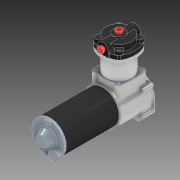
# Autodesk Inventor part: 215 Thomas Compressor
Saved by Autodesk Inventor 2022 (Build 260153000, 153)
## iProperties
Created: 2021-07-29
Part Number: 215 Thomas Compressor
Material: Generic
Document SubType Name: Modeling
Designer: kevin
Density: 1 g/cm^3
Appearance: Default
Author: kevin
Autodesk Inventor part; units mm, degrees
ref_plane "YZ Plane" through (0, 0, 0) normal (1, 0, 0) x (0, 1, 0)
sketch "Sketch37" plane through (0, 0, 0) normal (1, 0, 0) x (0, 1, 0)
  line L0 (0, 0) -> (27.7812, 0)
  line L1 (27.7812, 0) -> (27.7812, 50.8)
  line L2 (27.7812, 50.8) -> (25.4, 50.8)
  line L3 (25.4, 50.8) -> (25.4, 136.271)
  line L4 (25.4, 136.271) -> (15.5575, 136.271)
  line L5 (15.5575, 136.271) -> (15.5575, 138.811)
  line L6 (15.5575, 138.811) -> (12.7, 138.811)
  line L7 (12.7, 138.811) -> (8.2867, 146.431)
  line L8 (8.2867, 146.431) -> (0, 146.431)
  line L9 (0, 146.431) -> (0, 0)
  line L10 (0, 133.096) -> (25.4, 133.096)
  line L11 (25.4, 50.8) -> (0, 50.8)
  dimension "d151" = 27.7812
  dimension "d152" = 25.4
  dimension "d153" = 15.5575
  dimension "d154" = 12.7
  dimension "d156" = 8.2867
  dimension "d157" = 85.471
  dimension "d158" = 50.8
  dimension "d159" = 2.54
  dimension "d160" = 7.62
  dimension "d172" = 3.175
  constraints: 24 end point, 8 perpendicular, 3 point on line, 1 collinear, 1 horizontal, 1 parallel
  measures "d151" distance between parallel lines of L9 L1
  measures "d152" distance between parallel lines of L9 L3
  measures "d153" distance between parallel lines of L9 L5
  measures "d154" distance from line of L9 L6.end
  measures "d156" distance of L7.end L8.end
  measures "d157" distance of L2.end L3.end
  measures "d158" distance of L0.end L1.end
  measures "d159" distance of L4.end L5.end
  measures "d160" distance between parallel lines of L6 L8
  measures "d172" distance between parallel lines of L10 L4
revolve "Revolution1" add sketch "Sketch37" angle 360 about axis through (0, 0, 146.431) along (0, 0, -1) contours L9 L11 L2 L1 L0
sketch "Sketch38" plane through (0, 0, 0) normal (0, 1, 0) x (-1, 0, 0)
  line L0 (-17.4625, 42.8625) -> (17.4625, 42.8625) construction
  line L1 (17.4625, 42.8625) -> (17.4625, 7.9375) construction
  line L2 (17.4625, 7.9375) -> (-17.4625, 7.9375)
  line L3 (-17.4625, 7.9375) -> (-17.4625, 42.8625) construction
  line L4 (-17.4625, 42.8625) -> (17.4625, 7.9375) construction
  line L5 (17.4625, 42.8625) -> (-17.4625, 7.9375) construction
  circle A0 centre (0, 25.4) radius 20.6375
  line L6 (17.4625, 42.8625) -> (17.4625, 7.9375) construction
  line L7 (12.3825, 42.8625) -> (12.3825, 7.9375) construction
  line L8 (22.5425, 7.9375) -> (22.5425, 42.8625)
  arc A1 (22.5425, 42.8625) -> (12.3825, 42.8625) centre (17.4625, 42.8625) ccw
  arc A2 (12.3825, 7.9375) -> (22.5425, 7.9375) centre (17.4625, 7.9375) ccw
  line L9 (-17.4625, 7.9375) -> (-17.4625, 42.8625) construction
  line L10 (-12.3825, 7.9375) -> (-12.3825, 42.8625) construction
  line L11 (-22.5425, 42.8625) -> (-22.5425, 7.9375)
  arc A3 (-22.5425, 7.9375) -> (-12.3825, 7.9375) centre (-17.4625, 7.9375) ccw
  arc A4 (-12.3825, 42.8625) -> (-22.5425, 42.8625) centre (-17.4625, 42.8625) ccw
  line L12 (-27.7813, 50.8) -> (27.7813, 50.8) construction
  line L13 (17.4625, 42.8625) -> (13.056, 45.3901) construction
  line L14 (-13.056, 45.3901) -> (13.056, 45.3901) construction
  line L15 (-17.4625, 42.8625) -> (-13.056, 45.3901) construction
  arc A5 (13.056, 45.3901) -> (-13.056, 45.3901) centre (0, 12.9973) ccw
  line L16 (27.7812, 50.8) -> (27.7812, 0) construction
  line L17 (27.7812, 25.4) -> (-27.7812, 25.4) construction
  line L18 (-27.7812, 50.8) -> (-27.7812, 0) construction
  circle A6 centre (-17.4625, 42.8625) radius 1.7272
  circle A7 centre (-17.4625, 7.9375) radius 1.7272
  circle A8 centre (17.4625, 7.9375) radius 1.7272
  circle A9 centre (17.4625, 42.8625) radius 1.7272
  arc A10 (-13.056, 5.4099) -> (13.056, 5.4099) centre (0, 37.8027) ccw
  point P0 (0, 0)
  point P1 (17.4625, 25.4)
  point P2 (-17.4625, 25.4)
  point P3 (0, 25.4)
  point P4 (12.3825, 7.9375)
  point P5 (13.056, 45.3901)
  point P6 (-13.056, 45.3901)
  point P7 (-12.3825, 7.9375)
  point P8 (-10.9985, 7.9375)
  point P9 (10.9985, 7.9375)
  point P10 (13.056, 5.4099)
  dimension "d162" = 34.925
  dimension "d163" = 41.275
  dimension "d164" = 10.16
  dimension "d165" = 25.4
  dimension "d166" = 5.08
  dimension "d167" = 34.925
  dimension "d168" = 23.876
  dimension "d169" = 3.4544
  constraints: 36 end point, 12 point on circle, 11 centre point, 8 equal length, 8 midpoint, 8 tangent, 5 coincident, 4 equal radius, 3 symmetric about line, 2 horizontal, 1 perpendicular, 1 other
  measures "d162" distance of L0.end L1.end
  measures "d163" diameter of A0
  measures "d164" distance between parallel lines of L11 L10
  measures "d165" distance from line of A0.centre L12
  measures "d166" distance of L0.end L13.end
  measures "d167" radius of A5
  measures "d168" distance of point (0, 25.4) L13.end
  measures "d169" diameter of A8
extrude "Extrusion4" add sketch "Sketch38" along normal blind 35.8775
revolve "Revolution2" add sketch "Sketch37" angle 360 about axis through (0, 0, 146.431) along (0, 0, -1) separate body contours L9 L8 L7 L6 L5 L4 L3 L10
revolve "Revolution3" add sketch "Sketch37" angle 360 about axis through (0, 0, 146.431) along (0, 0, -1) separate body contours L9 L10 L3 L11
sketch "Sketch39" plane through (0, 35.8775, 0) normal (0, 1, 0) x (1, 0, 0)
  circle A0 centre (17.4625, -7.9375) radius 1.7272 construction
  circle A1 centre (-17.4625, -42.8625) radius 1.7272 construction
  line L0 (17.4625, -7.9375) -> (-17.4625, -42.8625) construction
  circle A2 centre (0, -25.4) radius 20.6375
  point P0 (0, 0)
  dimension "d175" = 41.275
  constraints: 2 end point, 1 centre point, 1 midpoint
  measures "d175" diameter of A2
extrude "Extrusion5" add sketch "Sketch39" along normal blind 28.575 separate body
sketch "Sketch40" plane through (0, 64.4525, 25.4) normal (0, 1, 0) x (1, 0, 0)
  arc A0 (20.5522, -18.5984) -> (20.5522, 18.5984) centre (-12.7, 0) ccw
  arc A1 (20.5522, 18.5984) -> (18.5984, 20.5522) centre (16.1186, 16.1186) ccw
  arc A2 (18.5984, 20.5522) -> (-18.5984, 20.5522) centre (0, -12.7) ccw
  arc A3 (-18.5984, 20.5522) -> (-20.5522, 18.5984) centre (-16.1186, 16.1186) ccw
  arc A4 (-20.5522, 18.5984) -> (-20.5522, -18.5984) centre (12.7, 0) ccw
  arc A5 (-20.5522, -18.5984) -> (-18.5984, -20.5522) centre (-16.1186, -16.1186) ccw
  arc A6 (-18.5984, -20.5522) -> (18.5984, -20.5522) centre (0, 12.7) ccw
  arc A7 (18.5984, -20.5522) -> (20.5522, -18.5984) centre (16.1186, -16.1186) ccw
  circle A8 centre (0, 0) radius 20.6375
  circle A9 centre (17.4625, -17.4625) radius 1.7272 projected
  circle A10 centre (-17.4625, -17.4625) radius 1.7272 projected
  circle A11 centre (-17.4625, 17.4625) radius 1.7272 projected
  circle A12 centre (17.4625, 17.4625) radius 1.7272 projected
  line L0 (0, -12.7) -> (0, 0) construction
  line L1 (0, 0) -> (-12.7, 0) construction
  line L2 (0, 0) -> (12.7, 0) construction
  line L3 (0, 12.7) -> (0, 0) construction
  line L4 (-16.1186, -16.1186) -> (0, 0) construction
  line L5 (-16.1186, 16.1186) -> (0, 0) construction
  line L6 (16.1186, -16.1186) -> (0, 0) construction
  line L7 (0, 0) -> (16.1186, 16.1186) construction
  line L8 (-22.5425, 17.4625) -> (-22.5425, -17.4625) construction
  line L9 (-22.5425, 0) -> (22.5425, 0) construction
  line L10 (22.5425, 17.4625) -> (22.5425, -17.4625) construction
  line L11 (0, 25.4) -> (0, -25.4) construction
  line L12 (27.7813, -25.4) -> (-27.7812, -25.4) construction
  line L13 (27.7813, 25.4) -> (-27.7812, 25.4) construction
  dimension "d179" = 5.08
  dimension "d180" = 12.7
  dimension "d181" = 45
  dimension "d182" = 41.275
  dimension "d197" = 50.8
  constraints: 20 end point, 16 point on circle, 9 centre point, 6 equal radius, 5 tangent, 4 midpoint, 3 equal length, 3 perpendicular, 2 vertical, 1 collinear, 1 horizontal
  measures "d179" radius of A1
  measures "d180" distance of L0.end L1.end
  measures "d181" angle of L0 L4
  measures "d182" diameter of A8
  measures "d197" distance of L11.start L11.end
extrude "Extrusion6" add sketch "Sketch40" along normal blind 6.35 separate body contours A7 A6 A5 A4 A3 A2 A1 A0 | A8
sketch "Sketch41" plane through (0, 70.8025, 25.4) normal (0, 1, 0) x (1, 0, 0)
  circle A0 centre (0, 0) radius 20.6375 construction
  circle A1 centre (0, 0) radius 20.0025
  point P0 (0, 25.4)
  dimension "d185" = 40.005
  constraints: 1 centre point, 1 coincident
  measures "d185" diameter of A1
extrude "Extrusion7" add sketch "Sketch41" along normal blind 9.525 bodies 5
sketch "Sketch42" plane through (0, 80.3275, 25.4) normal (0, 1, 0) x (1, 0, 0)
  circle A0 centre (0, 0) radius 20.0025 projected
  circle A1 centre (0, 0) radius 9.144
  point P0 (0, 25.4)
  dimension "d188" = 18.288
  constraints: 1 centre point, 1 coincident
  measures "d188" diameter of A1
extrude "Extrusion8" add sketch "Sketch42" along normal blind 2.54 contours A1 bodies 5
sketch "Sketch43" plane through (0, 70.8025, 25.4) normal (0, 1, 0) x (1, 0, 0)
  line L0 (16.1186, -16.1186) -> (-16.1186, 16.1186) construction
  circle A0 centre (0, 0) radius 9.144 projected
  line L1 (19.7107, -12.5265) -> (-12.5265, 19.7107)
  line L2 (-19.7107, 12.5265) -> (12.5265, -19.7107)
  arc A1 (12.5265, -19.7107) -> (19.7107, -12.5265) centre (16.1186, -16.1186) ccw
  arc A2 (-12.5265, 19.7107) -> (-19.7107, 12.5265) centre (-16.1186, 16.1186) ccw
  line L3 (16.1186, 16.1186) -> (-16.1186, -16.1186) construction
  line L4 (19.7107, 12.5265) -> (-12.5265, -19.7107)
  line L5 (-19.7107, -12.5265) -> (12.5265, 19.7107)
  arc A3 (19.7107, 12.5265) -> (12.5265, 19.7107) centre (16.1186, 16.1186) ccw
  arc A4 (-19.7107, -12.5265) -> (-12.5265, -19.7107) centre (-16.1186, -16.1186) ccw
  arc A5 (-20.5522, -18.5984) -> (-18.5984, -20.5522) centre (-16.1186, -16.1186) ccw projected
  line L6 (-22.5425, 0) -> (22.5425, 0) construction
  circle A6 centre (-17.4625, -17.4625) radius 1.7272 projected
  circle A7 centre (-17.4625, 17.4625) radius 1.7272 projected
  circle A8 centre (17.4625, 17.4625) radius 1.7272 projected
  circle A9 centre (17.4625, -17.4625) radius 1.7272 projected
  circle A10 centre (0, 0) radius 9.144 projected
  circle A11 centre (0, 0) radius 20.0025 projected
  line L7 (22.5425, -17.4625) -> (22.5425, 17.4625) construction
  line L8 (-22.5425, 17.4625) -> (-22.5425, -17.4625) construction
  point P0 (0, 25.4)
  point P1 (-10.0881, -17.2723)
  point P2 (-17.2723, -10.0881)
  point P3 (-17.2723, 10.0881)
  point P4 (-10.0881, 17.2723)
  point P5 (10.0881, 17.2723)
  point P6 (17.2723, 10.0881)
  point P7 (17.2723, -10.0881)
  point P8 (10.0881, -17.2723)
  dimension "d191" = 10.16
  dimension "d192" = 45
  constraints: 18 end point, 9 tangent, 8 point on circle, 4 centre point, 4 midpoint, 2 parallel, 2 perpendicular, 1 equal radius
  measures "d191" distance between parallel lines of L4 L5
  measures "d192" angle of L6 L5
extrude "Extrusion9" add sketch "Sketch43" along normal blind 5.334 contours A11 L5 A3 L4 | L1 A1 L2 A11 | A11 L2 A2 L1 | L4 A4 L5 A11 bodies 5
ref_plane "Work Plane1" through (0, 64.4525, 0) normal (0, 0, -1) x (-1, 0, 0)
sketch "Sketch44" plane through (0, 64.4525, 0) normal (0, 0, -1) x (-1, 0, 0)
  line L0 (20.6375, 0) -> (-20.6375, 0) projected
  line L1 (0, 0) -> (0, 8.89) construction
  line L2 (8.89, 0) -> (8.89, 8.89)
  line L3 (-8.89, 8.89) -> (-8.89, 0)
  arc A0 (-8.89, 0) -> (8.89, 0) centre (0, 0) ccw
  arc A1 (8.89, 8.89) -> (-8.89, 8.89) centre (0, 8.89) ccw
  line L4 (9.144, 18.415) -> (-9.144, 18.415) projected
  point P0 (0, -64.4525)
  point P1 (0, 4.445)
  dimension "d195" = 17.78
  dimension "d196" = 9.525
  constraints: 8 end point, 4 point on circle, 4 tangent, 2 centre point, 2 midpoint, 1 parallel, 1 vertical
  measures "d195" distance between parallel lines of L2 L3
  measures "d196" distance from line of L4 L1.end
extrude "Extrusion10" add sketch "Sketch44" against normal blind 50.8 contours L0 L3 A1 L2 bodies 5
move or copy body "Move Body1" bodies to move or copy 5 copy no translate (0, 4.7625, 0)
sketch "Sketch45" plane through (12.7, 69.215, 25.4) normal (0, -1, 0) x (1, 0, 0)
  circle A0 centre (4.7625, 17.4625) radius 1.7272 projected
  circle A1 centre (4.7625, -17.4625) radius 1.7272 projected
  arc A2 (-21.59, 24.3483) -> (-31.2984, 20.5522) centre (-12.7, -12.7) ccw projected
  arc A3 (-31.2984, 20.5522) -> (-33.2522, 18.5984) centre (-28.8186, 16.1186) ccw projected
  arc A4 (-33.2522, 18.5984) -> (-33.2522, -18.5984) centre (0, 0) ccw projected
  arc A5 (-33.2522, -18.5984) -> (-31.2984, -20.5522) centre (-28.8186, -16.1186) ccw projected
  arc A6 (-31.2984, -20.5522) -> (-21.59, -24.3483) centre (-12.7, 12.7) ccw projected
  line L0 (-21.59, -25.4) -> (-21.59, -24.3483) projected
  line L1 (-3.81, -25.4) -> (-21.59, -25.4) projected
  line L2 (-3.81, -25.4) -> (-3.81, -24.3483) projected
  arc A7 (-3.81, -24.3483) -> (5.8984, -20.5522) centre (-12.7, 12.7) ccw projected
  arc A8 (5.8984, -20.5522) -> (7.8522, -18.5984) centre (3.4186, -16.1186) ccw projected
  arc A9 (7.8522, -18.5984) -> (7.8522, 18.5984) centre (-25.4, 0) ccw projected
  arc A10 (7.8522, 18.5984) -> (5.8984, 20.5522) centre (3.4186, 16.1186) ccw projected
  arc A11 (5.8984, 20.5522) -> (-3.81, 24.3483) centre (-12.7, -12.7) ccw projected
  line L3 (-3.81, 24.3483) -> (-3.81, 25.4) projected
  line L4 (-21.59, 25.4) -> (-3.81, 25.4) projected
  line L5 (-21.59, 24.3483) -> (-21.59, 25.4) projected
  circle A12 centre (-30.1625, -17.4625) radius 1.7272 projected
  circle A13 centre (-30.1625, 17.4625) radius 1.7272 projected
  line L6 (-21.59, 24.3483) -> (-21.59, 17.9184) projected
  arc A14 (-3.81, 24.3483) -> (-21.59, 24.3483) centre (-12.7, -12.7) ccw
  line L7 (0, 0) -> (-25.4, 0) construction
  arc A15 (-21.59, -24.3483) -> (-3.81, -24.3483) centre (-12.7, 12.7) ccw
  point P0 (-12.7, -25.4)
  constraints: 4 point on circle, 2 centre point, 2 end point, 1 concentric, 1 horizontal, 1 symmetric about line, 1 other
extrude "Extrusion11" add sketch "Sketch45" along normal up to surface (4.7625 mm away) separate body contours A14 A11 A10 A9 A8 A7 A15 A6 A5 A4 A3 A2
sketch "Sketch46" plane through (0, 87.63, 25.4) normal (0, 1, 0) x (1, 0, 0)
  arc A0 (5.4993, -7.3055) -> (5.4993, 7.3055) centre (0, 0) ccw projected
  circle A1 centre (0, 0) radius 3.175
  circle A2 centre (0, 0) radius 3.937
  point P0 (0, 25.4)
  dimension "d205" = 6.35
  dimension "d206" = 0.762
  constraints: 2 centre point, 1 coincident
  measures "d205" diameter of A1
  measures "d206" radial gap between concentric circles of A1 A2
extrude "Extrusion12" add sketch "Sketch46" along normal blind 3.175 separate body
sketch "Sketch47" plane through (0, 90.805, 25.4) normal (0, 1, 0) x (1, 0, 0)
  circle A0 centre (0, 0) radius 3.175 projected
  circle A1 centre (0, 0) radius 5.08
  point P0 (0, 25.4)
  dimension "d209" = 10.16
  constraints: 1 centre point, 1 coincident
  measures "d209" diameter of A1
extrude "Extrusion13" add sketch "Sketch47" along normal blind 0.7937 bodies 7
sketch "Sketch48" plane through (0, 78.105, 50.8) normal (0, 0, 1) x (1, 0, 0)
  arc A0 (8.89, 0) -> (-8.89, 0) centre (0, 0) ccw projected
  circle A1 centre (0, 0) radius 3.937
  circle A2 centre (0, 0) radius 3.175
  point P0 (0, -78.105)
  dimension "d212" = 7.874
  dimension "d213" = 6.35
  constraints: 2 centre point, 2 coincident
  measures "d212" diameter of A1
  measures "d213" diameter of A2
extrude "Extrusion14" add sketch "Sketch48" along normal blind 3.175 bodies 7
sketch "Sketch49" plane through (0, 78.105, 53.975) normal (0, 0, 1) x (1, 0, 0)
  circle A0 centre (0, 0) radius 3.175 projected
  circle A1 centre (0, 0) radius 5.08
  point P0 (0, -78.105)
  dimension "d216" = 10.16
  constraints: 1 centre point
  measures "d216" diameter of A1
extrude "Extrusion15" add sketch "Sketch49" along normal blind 0.7937 bodies 7
sketch "Sketch51" plane through (0, 0, 0) normal (0, 0, -1) x (-1, 0, 0)
  line L0 (25.7175, 16.8275) -> (-25.7175, 16.8275) construction
  line L1 (25.7175, 20.0025) -> (-25.7175, 20.0025)
  line L2 (-25.7175, 13.6525) -> (25.7175, 13.6525)
  arc A0 (25.7175, 13.6525) -> (25.7175, 20.0025) centre (25.7175, 16.8275) ccw
  arc A1 (-25.7175, 20.0025) -> (-25.7175, 13.6525) centre (-25.7175, 16.8275) ccw
  line L3 (13.056, 35.8775) -> (-13.056, 35.8775) construction
  line L4 (0, 35.8775) -> (0, 20.0025) construction
  line L5 (-25.7175, 13.6525) -> (-25.7175, 10.5075)
  circle A2 centre (0, 0) radius 27.7812 projected
  line L6 (25.7175, 13.6525) -> (25.7175, 10.5075)
  line L7 (-12.7, 27.94) -> (12.7, 27.94)
  line L8 (-12.7, 27.94) -> (-12.7, 24.7085)
  line L9 (13.056, 24.5222) -> (13.056, 35.8775) projected
  line L10 (12.7, 27.94) -> (12.7, 24.7085)
  line L11 (-25.7175, -21.9075) -> (25.7175, -21.9075)
  line L12 (25.7175, -18.7325) -> (-25.7175, -18.7325) construction
  line L13 (25.7175, -15.5575) -> (-25.7175, -15.5575)
  arc A3 (-25.7175, -15.5575) -> (-25.7175, -21.9075) centre (-25.7175, -18.7325) ccw
  arc A4 (25.7175, -21.9075) -> (25.7175, -15.5575) centre (25.7175, -18.7325) ccw
  line L14 (-25.7175, -15.5575) -> (-25.7175, -10.5075)
  line L15 (25.7175, -15.5575) -> (25.7175, -10.5075)
  line L16 (21.3176, -27.6225) -> (11.7926, -27.6225)
  line L17 (21.3176, -27.6225) -> (27.9626, -20.9776)
  line L18 (11.7926, -27.6225) -> (10.0643, -25.8942)
  line L19 (-21.3176, -27.6225) -> (-11.7926, -27.6225)
  line L20 (-21.3176, -27.6225) -> (-27.9626, -20.9776)
  line L21 (-11.7926, -27.6225) -> (-10.0643, -25.8942)
  point P0 (0, 0)
  point P1 (0, 16.8275)
  point P2 (0, 27.94)
  point P3 (0, -15.5575)
  point P4 (19.2795, 20.0025)
  point P5 (-19.2795, 20.0025)
  dimension "d219" = 51.435
  dimension "d220" = 6.35
  dimension "d221" = 15.875
  dimension "d222" = 25.4
  dimension "d223" = 7.9375
  dimension "d226" = 35.56
  dimension "d231" = 63.5
  dimension "d232" = 9.525
  dimension "d233" = 135
  constraints: 44 end point, 9 point on circle, 5 midpoint, 5 tangent, 4 centre point, 4 parallel, 4 symmetric about line, 4 vertical, 3 horizontal, 2 perpendicular, 21 other
  measures "d219" distance of L0.start L0.end
  measures "d220" distance between parallel lines of L1 L2
  measures "d221" distance of L4.start L4.end
  measures "d222" distance of L7.start L7.end
  measures "d223" distance between parallel lines of L7 L3
  measures "d226" distance of L2.start L11.start
  measures "d231" distance between parallel lines of L16 L3
  measures "d232" distance of L16.start L16.end
  measures "d233" angle of L16 L17
extrude "Extrusion16" add sketch "Sketch51" against normal blind 15.875 bodies 1
sketch "Sketch52" plane through (12.7, 27.94, 0) normal (0, 0, -1) x (-1, 0, 0)
  arc A0 (0, -3.2315) -> (-6.5795, -7.9375) centre (12.7, -27.94) ccw projected
  line L0 (-6.5795, -7.9375) -> (-13.0175, -7.9375) projected
  arc A1 (-13.0175, -7.9375) -> (-13.0175, -14.2875) centre (-13.0175, -11.1125) ccw projected
  line L1 (-13.0175, -14.2875) -> (-13.0175, -17.4325) projected
  arc A2 (-13.0175, -17.4325) -> (-13.0175, -38.4475) centre (12.7, -27.94) ccw projected
  line L2 (-13.0175, -38.4475) -> (-13.0175, -43.4975) projected
  arc A3 (-13.0175, -43.4975) -> (-15.2626, -48.9176) centre (-13.0175, -46.6725) ccw projected
  line L3 (-15.2626, -48.9176) -> (-8.6176, -55.5625) projected
  line L4 (-8.6176, -55.5625) -> (0.9074, -55.5625) projected
  line L5 (0.9074, -55.5625) -> (2.6357, -53.8342) projected
  arc A4 (2.6357, -53.8342) -> (22.7643, -53.8342) centre (12.7, -27.94) ccw projected
  line L6 (22.7643, -53.8342) -> (24.4926, -55.5625) projected
  line L7 (24.4926, -55.5625) -> (34.0176, -55.5625) projected
  line L8 (34.0176, -55.5625) -> (40.6626, -48.9176) projected
  arc A5 (40.6626, -48.9176) -> (38.4175, -43.4975) centre (38.4175, -46.6725) ccw projected
  line L9 (38.4175, -43.4975) -> (38.4175, -38.4475) projected
  arc A6 (38.4175, -38.4475) -> (38.4175, -17.4325) centre (12.7, -27.94) ccw projected
  line L10 (38.4175, -17.4325) -> (38.4175, -14.2875) projected
  arc A7 (38.4175, -14.2875) -> (38.4175, -7.9375) centre (38.4175, -11.1125) ccw projected
  line L11 (38.4175, -7.9375) -> (31.9795, -7.9375) projected
  arc A8 (31.9795, -7.9375) -> (25.4, -3.2315) centre (12.7, -27.94) ccw projected
  line L12 (25.4, -3.2315) -> (25.4, 0) projected
  line L13 (25.4, 0) -> (0, 0) projected
  line L14 (0, 0) -> (0, -3.2315) projected
  arc A9 (-13.0175, -43.4975) -> (-15.2626, -48.9176) centre (-13.0175, -46.6725) ccw projected
  arc A10 (-15.2626, -48.9176) -> (-13.7832, -49.7538) centre (-13.0175, -46.6725) ccw
  line L15 (-13.7832, -49.7538) -> (2.6357, -53.8342)
  line L16 (12.7, -27.94) -> (12.7, -55.7212) construction
  circle A11 centre (12.7, -27.94) radius 27.7813 construction
  arc A12 (39.1832, -49.7538) -> (40.6626, -48.9176) centre (38.4175, -46.6725) ccw
  line L17 (39.1832, -49.7538) -> (22.7643, -53.8342)
  arc A13 (-13.0175, -7.9375) -> (-13.0175, -14.2875) centre (-13.0175, -11.1125) ccw projected
  line L18 (-16.1925, -11.1125) -> (-16.1925, -46.6725)
  arc A14 (40.6626, -48.9176) -> (38.4175, -43.4975) centre (38.4175, -46.6725) ccw projected
  line L19 (41.5925, -46.6725) -> (41.5925, -11.1125)
  arc A15 (40.6626, -48.9176) -> (38.4175, -43.4975) centre (38.4175, -46.6725) ccw projected
  arc A16 (-13.0175, -7.9375) -> (-13.0175, -14.2875) centre (-13.0175, -11.1125) ccw projected
  point P0 (-16.1925, -11.1125)
  point P1 (-16.1925, -46.6725)
  constraints: 10 end point, 9 point on circle, 5 tangent, 2 centre point, 2 symmetric about line, 1 concentric, 1 vertical, 3 other
extrude "Extrusion17" add sketch "Sketch52" along normal blind 1.905 separate body contours L14 L13 L12 A8 L11 A7 L10 A6 L9 A5 A12 L17 A4 L15 A10 A3 L2 A2 L1 A1 L0 A0 | A1 L1 A2 L2 A3 L18 | L19 A5 L9 A6 L10 A7
sketch "Sketch53" plane through (12.7, 27.94, -1.905) normal (0, 0, -1) x (-1, 0, 0)
  circle A0 centre (12.7, -27.94) radius 25.4 construction
  arc A1 (0, -3.2315) -> (-6.5795, -7.9375) centre (12.7, -27.94) ccw construction
  line L0 (-16.1925, -11.1125) -> (-16.1925, -46.6725) construction
  arc A2 (-6.5795, -7.9375) -> (-16.1925, -30.5545) centre (15.22, -30.5545) ccw
  line L1 (41.5925, -46.6725) -> (41.5925, -11.1125) construction
  arc A3 (31.9795, -7.9375) -> (25.4, -3.2315) centre (12.7, -27.94) ccw construction
  arc A4 (41.5925, -30.5545) -> (31.9795, -7.9375) centre (10.18, -30.5545) ccw
  arc A5 (31.9795, -7.9375) -> (25.4, -3.2315) centre (12.7, -27.94) ccw construction
  line L2 (41.5925, -46.6725) -> (41.5925, -11.1125) construction
  arc A6 (0, -3.2315) -> (-6.5795, -7.9375) centre (12.7, -27.94) ccw construction
  line L3 (-16.1925, -11.1125) -> (-16.1925, -46.6725) construction
  arc A7 (-16.1925, -46.6725) -> (-13.7832, -49.7538) centre (-13.0175, -46.6725) ccw projected
  line L4 (-13.7832, -49.7538) -> (2.6357, -53.8342) projected
  arc A8 (2.6357, -53.8342) -> (22.7643, -53.8342) centre (12.7, -27.94) ccw projected
  line L5 (22.7643, -53.8342) -> (39.1832, -49.7538) projected
  arc A9 (39.1832, -49.7538) -> (41.5925, -46.6725) centre (38.4175, -46.6725) ccw projected
  line L6 (41.5925, -46.6725) -> (41.5925, -11.1125) projected
  arc A10 (41.5925, -11.1125) -> (38.4175, -7.9375) centre (38.4175, -11.1125) ccw projected
  line L7 (38.4175, -7.9375) -> (31.9795, -7.9375) projected
  arc A11 (31.9795, -7.9375) -> (25.4, -3.2315) centre (12.7, -27.94) ccw projected
  line L8 (25.4, -3.2315) -> (25.4, 0) projected
  line L9 (25.4, 0) -> (0, 0) projected
  line L10 (0, 0) -> (0, -3.2315) projected
  arc A12 (0, -3.2315) -> (-6.5795, -7.9375) centre (12.7, -27.94) ccw projected
  line L11 (-6.5795, -7.9375) -> (-13.0175, -7.9375) projected
  arc A13 (-13.0175, -7.9375) -> (-16.1925, -11.1125) centre (-13.0175, -11.1125) ccw projected
  line L12 (-16.1925, -11.1125) -> (-16.1925, -46.6725) projected
  point P0 (41.5925, -30.5545)
  point P1 (-16.1925, -30.5545)
  point P2 (-6.5795, -7.9375)
  constraints: 4 point on circle, 4 tangent, 2 centre point, 2 point on line
extrude "Extrusion18" cut sketch "Sketch53" against normal up to surface (1.905 mm away) contours A2 L12 A13 L11 | L7 A10 L6 A4 bodies 8
sketch "Sketch54" plane through (12.7, 27.94, -1.905) normal (0, 0, -1) x (-1, 0, 0)
  circle A0 centre (12.7, -27.94) radius 15.5575 projected
extrude "Extrusion19" add sketch "Sketch54" along normal blind 3.175 separate body
sketch "Sketch55" plane through (0, 0, -5.08) normal (0, 0, -1) x (-1, 0, 0)
  circle A0 centre (0, 0) radius 8.2867 projected
  point P0 (0, 0)
extrude "Extrusion20" cut sketch "Sketch55" against normal blind 0.7937 bodies 9
sketch "Sketch56" plane through (12.7, 27.94, -1.905) normal (0, 0, -1) x (-1, 0, 0)
  arc A0 (-16.1925, -46.6725) -> (-13.7832, -49.7538) centre (-13.0175, -46.6725) ccw construction
  arc A1 (39.1832, -49.7538) -> (41.5925, -46.6725) centre (38.4175, -46.6725) ccw construction
  circle A2 centre (12.7, -27.94) radius 8.2867 construction
  line L0 (12.7, -27.94) -> (12.7, -12.3825) construction
  circle A3 centre (12.7, -27.94) radius 15.5575 construction
  line L1 (12.7, -12.3825) -> (12.7, 0) construction
  line L2 (25.4, 0) -> (0, 0) construction
  circle A4 centre (12.7, -6.1912) radius 1.778
  circle A5 centre (-13.0175, -46.6725) radius 1.778
  circle A6 centre (38.4175, -46.6725) radius 1.778
  dimension "d244" = 3.556
  constraints: 4 end point, 3 centre point, 2 coincident, 2 equal radius, 2 midpoint, 1 collinear, 1 vertical alignment, 1 other
  measures "d244" diameter of A4
extrude "Extrusion21" cut sketch "Sketch56" against normal blind 12.7 bodies 8 1
sketch "Sketch57" plane through (0, 0, 136.271) normal (0, 0, 1) x (1, 0, 0)
  circle A0 centre (0, 0) radius 25.4 projected
  line L0 (17.8548, -18.0657) -> (14.7116, -14.9225) construction
  line L1 (12.2421, -23.6783) -> (9.0989, -20.5352)
  line L2 (20.3243, -9.3098) -> (23.4674, -12.453)
  arc A1 (12.2421, -23.6783) -> (23.4674, -12.453) centre (17.8548, -18.0657) ccw
  arc A2 (20.3243, -9.3098) -> (9.0989, -20.5352) centre (14.7116, -14.9225) ccw
  circle A3 centre (0, 0) radius 8.2867 projected
  line L3 (13.056, 35.8775) -> (-13.056, 35.8775) projected
  point P0 (16.2832, -16.4941)
  point P1 (11.3078, -22.7441)
  point P2 (22.6025, -11.5881)
  dimension "d247" = 15.875
  dimension "d248" = 20.955
  dimension "d249" = 45
  dimension "d250" = 50.8
  constraints: 8 end point, 4 point on circle, 4 tangent, 2 centre point, 1 midpoint, 1 parallel, 2 other
  measures "d247" distance between parallel lines of L2 L1
  measures "d248" distance of L0.end A3.centre
  measures "d249" angle of L3 L2
  measures "d250" distance from line of L3 L0.end
extrude "Extrusion22" add sketch "Sketch57" along normal blind 6.35 contours L1 A2 L2 A0 picked at (15.1048, -14.8713) bodies 2
ref_plane "Work Plane4" through (18.7903, -19.024, 136.271) normal (0.7027227, -0.7114638, 0) x (0, 0, 1)
ref_plane "Work Plane2" through (22.6025, -11.5881, 136.271) normal (0.8898641, -0.4562257, 0) x (0.4562257, 0.8898641, 0)
ref_plane "Work Plane3" through (11.3078, -22.7441, 136.271) normal (0.4451907, -0.8954358, 0) x (0.8954358, 0.4451907, 0)
sketch "Sketch58" plane through (18.7903, -19.024, 136.271) normal (0.7027227, -0.7114638, 0) x (0, 0, 1)
  line L0 (6.35, -7.9177) -> (6.35, 7.957) construction
  line L1 (6.35, 0.0196) -> (0, 0) construction
  line L2 (0, 15.5575) -> (0, -15.5575) construction
  line L3 (3.175, 0.0098) -> (3.175, -2.5302) construction
  line L4 (3.175, 0.0098) -> (3.175, 2.5498) construction
  circle A0 centre (3.175, -2.5302) radius 2.2479
  circle A1 centre (3.175, 2.5498) radius 2.2479
  point P0 (-136.271, 0)
  point P1 (0, 4.9629)
  point P2 (0, -4.9353)
  point P3 (3.175, 0.0098)
  dimension "d253" = 5.08
  dimension "d254" = 4.4958
  constraints: 6 end point, 3 midpoint, 2 centre point, 2 coincident, 2 vertical, 1 collinear, 1 equal radius
  measures "d253" distance of L4.end L3.end
  measures "d254" diameter of A0
extrude "Extrusion23" cut sketch "Sketch58" against normal blind 6.35 bodies 2
sketch "Sketch59" plane through (16.1281, -12.7282, 139.446) normal (0.7027227, -0.7114638, 0) x (0.7114638, 0.7027227, 0)
  spline S0 degree 2 poles (0, 2.2479) (-3.8935, 2.2479) (-1.9467, -1.124) (0, -4.4958) (1.9467, -1.124) (3.8935, 2.2479) (0, 2.2479) knots 0 0 0 0.333333 0.333333 0.666667 0.666667 1 1 1 weights 1 0.5 1 0.5 1 0.5 1 projected
  spline S1 degree 2 poles (-5.08, 2.2479) (-8.9735, 2.2479) (-7.0267, -1.124) (-5.08, -4.4958) (-3.1333, -1.124) (-1.1865, 2.2479) (-5.08, 2.2479) knots 0 0 0 0.333333 0.333333 0.666667 0.666667 1 1 1 weights 1 0.5 1 0.5 1 0.5 1 projected
  circle A0 centre (0, 0) radius 1.27
  circle A1 centre (0, 0) radius 2.2479 projected
  circle A2 centre (-5.08, 0) radius 1.27
  circle A3 centre (-5.08, 0) radius 2.2479 projected
  point P0 (-2.5302, -139.446)
  dimension "d257" = 2.54
  constraints: 2 centre point, 2 horizontal alignment, 1 equal radius, 4 other
  measures "d257" diameter of A0
extrude "Extrusion24" add sketch "Sketch59" along normal blind 6.35 separate body
sketch "Sketch61" plane through (0, 0, 136.271) normal (0, 0, 1) x (1, 0, 0)
  line L0 (0, 0) -> (0, 19.05) construction
  circle A0 centre (0, 19.05) radius 1.7272
  line L1 (-4.7625, 23.8125) -> (4.7625, 23.8125)
  line L2 (4.7625, 23.8125) -> (4.7625, 0)
  line L3 (4.7625, 0) -> (-4.7625, 0)
  line L4 (-4.7625, 0) -> (-4.7625, 23.8125)
  arc A1 (13.8792, -7.0288) -> (6.8305, -13.9778) centre (0, 0) ccw projected
  line L5 (0, 0) -> (0, -19.05) construction
  circle A2 centre (0, -19.05) radius 1.7272
  line L6 (4.7625, -23.8125) -> (-4.7625, -23.8125)
  line L7 (-4.7625, -23.8125) -> (-4.7625, 0)
  line L8 (4.7625, 0) -> (4.7625, -23.8125)
  point P0 (-4.7625, 14.8106)
  point P1 (4.7625, 14.8106)
  point P2 (4.7625, -14.8106)
  point P3 (-4.7625, -14.8106)
  dimension "d260" = 19.05
  dimension "d261" = 3.4544
  dimension "d262" = 9.525
  dimension "d263" = 4.7625
  dimension "d266" = 360
  constraints: 18 end point, 4 coincident, 2 centre point, 2 parallel, 1 horizontal, 1 midpoint, 1 perpendicular, 1 vertical, 23 other
  measures "d260" distance of L0.start L0.end
  measures "d261" diameter of A0
  measures "d262" distance of L1.start L1.end
  measures "d263" distance from line of L1 A0.centre
extrude "Extrusion25" add sketch "Sketch61" along normal blind 1.905 contours L1 L2 A1 L4 | A1 L8 L6 L7 bodies 2
fillet "Fillet2" radius 0.7937 4 edges at (-4.7625, 23.8125, 137.2235) (4.7625, 23.8125, 137.2235) (-4.7625, -23.8125, 137.2235) (4.7625, -23.8125, 137.2235)
body "Solid9"
body "Solid10"
body "Solid11"
body "Solid12"
